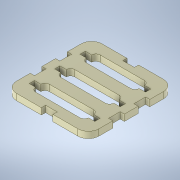
# Autodesk Inventor part: Крепление РБАСУ
Saved by Autodesk Inventor 2022 (Build 260153000, 153)
## iProperties
Created: 2022-05-03
Part Number: Крепление РБАСУ
Material: Пластик АБС
Document SubType Name: Modeling
Designer: Кочетов.А.И.
Density: 1.06 g/cm^3
Appearance: Гладкий — пепельный
Author: Кочетов.А.И.
Autodesk Inventor part; units mm, degrees
ref_plane "YZ Plane" through (0, 0, 0) normal (1, 0, 0) x (0, 1, 0)
ref_plane "XZ Plane" through (0, 0, 0) normal (0, 1, 0) x (-1, 0, 0)
ref_plane "XY Plane" through (0, 0, 0) normal (0, 0, 1) x (1, 0, 0)
sketch "Эскиз1" plane through (0, 0, 0) normal (0, 1, 0) x (-1, 0, 0)
  line L0 (19.5, 0) -> (12.5, 0)
  line L1 (12.5, 0) -> (12.5, -40.5)
  line L2 (12.5, -40.5) -> (19.5, -40.5)
  line L3 (19.5, -40.5) -> (19.5, 0)
  line L4 (-12.5, 0) -> (-19.5, 0)
  line L5 (-19.5, 0) -> (-19.5, -40.5)
  line L6 (-19.5, -40.5) -> (-12.5, -40.5)
  line L7 (-12.5, -40.5) -> (-12.5, 0)
  line L8 (0, 0) -> (0, -102.7933) construction
  line L9 (12.5, -7) -> (15.5, -7)
  line L10 (15.5, -7) -> (15.5, -9.5)
  line L11 (15.5, -9.5) -> (12.5, -9.5)
  line L12 (12.5, -9.5) -> (12.5, -7)
  line L13 (-12.5, -7) -> (-15.5, -7)
  line L14 (-15.5, -7) -> (-15.5, -9.5)
  line L15 (-15.5, -9.5) -> (-12.5, -9.5)
  line L16 (-12.5, -9.5) -> (-12.5, -7)
  line L17 (15.5, -21.5) -> (12.5, -21.5)
  line L18 (12.5, -19) -> (15.5, -19)
  line L19 (15.5, -19) -> (15.5, -21.5)
  line L20 (12.5, -21.5) -> (12.5, -19)
  line L21 (-15.5, -21.5) -> (-12.5, -21.5)
  line L22 (-15.5, -19) -> (-15.5, -21.5)
  line L23 (-12.5, -19) -> (-15.5, -19)
  line L24 (-12.5, -21.5) -> (-12.5, -19)
  line L25 (15.5, -33.5) -> (12.5, -33.5)
  line L26 (12.5, -31) -> (15.5, -31)
  line L27 (15.5, -31) -> (15.5, -33.5)
  line L28 (12.5, -33.5) -> (12.5, -31)
  line L29 (-15.5, -33.5) -> (-12.5, -33.5)
  line L30 (-15.5, -31) -> (-15.5, -33.5)
  line L31 (-12.5, -31) -> (-15.5, -31)
  line L32 (-12.5, -33.5) -> (-12.5, -31)
  line L33 (19.5, 0) -> (-19.5, 0)
  line L34 (-12.5, -5) -> (12.5, -5)
  line L35 (-19.5, -40.5) -> (19.5, -40.5)
  line L36 (12.5, -35.5) -> (-12.5, -35.5)
  line L37 (12.5, -11.5) -> (-12.5, -11.5)
  line L38 (-12.5, -11.5) -> (-12.5, -17)
  line L39 (-12.5, -17) -> (12.5, -17)
  line L40 (12.5, -17) -> (12.5, -11.5)
  line L41 (12.5, -23.5) -> (-12.5, -23.5)
  line L42 (-12.5, -23.5) -> (-12.5, -29)
  line L43 (-12.5, -29) -> (12.5, -29)
  line L44 (12.5, -29) -> (12.5, -23.5)
  line L45 (19.5, -11.5) -> (17.5, -11.5)
  line L46 (17.5, -11.5) -> (17.5, -17)
  line L47 (17.5, -17) -> (19.5, -17)
  line L48 (19.5, -17) -> (19.5, -11.5)
  line L49 (19.5, -23.5) -> (17.5, -23.5)
  line L50 (17.5, -23.5) -> (17.5, -29)
  line L51 (17.5, -29) -> (19.5, -29)
  line L52 (19.5, -29) -> (19.5, -23.5)
  line L53 (-19.5, -11.5) -> (-17.5, -11.5)
  line L54 (-17.5, -11.5) -> (-17.5, -17)
  line L55 (-17.5, -17) -> (-19.5, -17)
  line L56 (-19.5, -17) -> (-19.5, -11.5)
  line L57 (-19.5, -23.5) -> (-17.5, -23.5)
  line L58 (-17.5, -23.5) -> (-17.5, -29)
  line L59 (-17.5, -29) -> (-19.5, -29)
  line L60 (-19.5, -29) -> (-19.5, -23.5)
  line L61 (2.75, 0) -> (-2.75, 0)
  line L62 (-2.75, 0) -> (-2.75, -2)
  line L63 (-2.75, -2) -> (2.75, -2)
  line L64 (2.75, -2) -> (2.75, 0)
  line L65 (2.75, -40.5) -> (-2.75, -40.5)
  line L66 (-2.75, -40.5) -> (-2.75, -38.5)
  line L67 (-2.75, -38.5) -> (2.75, -38.5)
  line L68 (2.75, -38.5) -> (2.75, -40.5)
  point P0 (-12.5, -40.5)
  point P1 (-12.5, -33.5)
  point P2 (-12.5, -31)
  point P3 (-12.5, -21.5)
  point P4 (-12.5, -19)
  point P5 (-12.5, -9.5)
  point P6 (12.5, -9.5)
  point P7 (12.5, -19)
  point P8 (12.5, -21.5)
  point P9 (12.5, -31)
  point P10 (12.5, -33.5)
  point P11 (12.5, -29)
  point P12 (12.5, -17)
  point P13 (-12.5, -11.5)
  point P14 (18.5, -17)
  point P15 (18.5, -11.5)
  point P16 (-18.5, -11.5)
  point P17 (-18.5, -17)
  point P18 (-18.5, -23.5)
  point P19 (18.5, -23.5)
  point P20 (-19.5, -17)
  point P21 (-19.5, -29)
  point P22 (19.5, -17)
  dimension "d0" = 2.5
  dimension "d1" = 3
  dimension "d4" = 12
  dimension "d9" = 31
  dimension "d10" = 4
  dimension "d11" = 5
  dimension "d12" = 5
  dimension "d14" = 2
  dimension "d17" = 2
  dimension "d18" = 2
  dimension "d19" = 2
  dimension "d20" = 2
  dimension "d21" = 2
  dimension "d24" = 2
  dimension "d25" = 2
  dimension "d26" = 5.5
  constraints: 138 end point, 34 point on line, 24 parallel, 15 perpendicular, 12 horizontal, 6 midpoint, 3 equal length, 2 vertical, 1 collinear, 1 horizontal alignment, 37 other
  measures "d0" distance of L9.end L10.end
  measures "d1" distance of L10.end L11.end
  measures "d4" distance of L10.end L17.start
  measures "d9" distance between parallel lines of L22 L19
  measures "d10" distance between parallel lines of L3 L27
  measures "d11" distance between parallel lines of L33 L34
  measures "d12" distance between parallel lines of L35 L36
  measures "d14" distance between parallel lines of L36 L25
  measures "d17" distance between parallel lines of L9 L34
  measures "d18" distance between parallel lines of L43 L26
  measures "d19" distance between parallel lines of L17 L41
  measures "d20" distance between parallel lines of L39 L18
  measures "d21" distance between parallel lines of L11 L37
  measures "d24" distance between parallel lines of L3 L50
  measures "d25" distance of L61.end L62.end
  measures "d26" distance between parallel lines of L64 L62
extrude "Выдавливание1" add sketch "Эскиз1" along normal blind 3 contours L3 L45 L46 L47 L49 L50 L51 L2 L1 L25 L27 L26 L17 L19 L18 L11 L10 L9 L0 | L1 L34 L7 L33 L62 L63 L64 | L7 L13 L14 L15 L23 L22 L21 L31 L30 L29 L6 L5 L59 L58 L57 L55 L54 L53 L4 | L1 L39 L7 L37 | L35 L68 L67 L66 L7 L36 L1 | L1 L43 L7 L41
fillet "Сопряжение1" radius 2 12 edges at (12.5, 1.5, -5) (-12.5, 1.5, -5) (-12.5, 1.5, -11.5) (12.5, 1.5, -11.5) (12.5, 1.5, -23.5) (12.5, 1.5, -35.5) (12.5, 1.5, -17) (12.5, 1.5, -29) (-12.5, 1.5, -17) (-12.5, 1.5, -23.5) (-12.5, 1.5, -35.5) (-12.5, 1.5, -29)
fillet "Сопряжение2" radius 5 4 edges at (-19.5, 1.5, 0) (19.5, 1.5, 0) (19.5, 1.5, -40.5) (-19.5, 1.5, -40.5)
equation "\"d12\" = d11"
